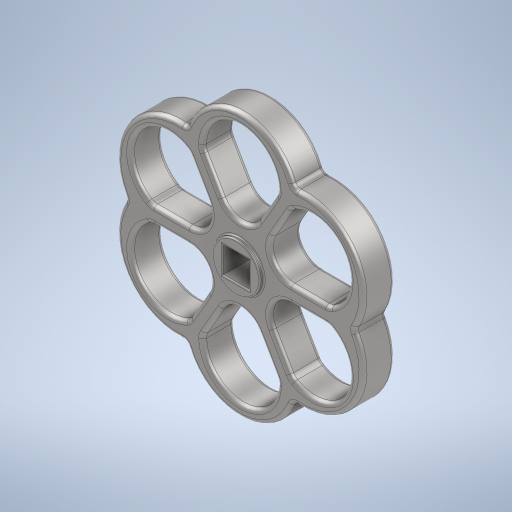
# Autodesk Inventor part: cover 2
Saved by Autodesk Inventor 2024 (Build 280153000, 153)
## iProperties
Created: 2024-04-01
Part Number: cover 2
Material: Generic
Document SubType Name: Modeling
Designer: MSI-C
Density: 1 g/cm^3
Appearance: Stainless - Brushed
Author: MSI-C
Autodesk Inventor part; units mm, degrees
ref_plane "YZ Plane" through (0, 0, 0) normal (1, 0, 0) x (0, 1, 0)
ref_plane "XZ Plane" through (0, 0, 0) normal (0, 1, 0) x (-1, 0, 0)
ref_plane "XY Plane" through (0, 0, 0) normal (0, 0, 1) x (1, 0, 0)
sketch "Sketch1" plane through (0, 0, 0) normal (0, 0, 1) x (1, 0, 0)
  line L0 (-42.5, 0) -> (42.5, 0) construction
  line L1 (0, 0) -> (20, 34.641) construction
  line L2 (0, 0) -> (-20, 34.641) construction
  line L3 (0, 49.3564) -> (0, -48.6436) construction
  arc A0 (19.9086, 34.4827) -> (-20, 34.641) centre (-0.0697, 28.5022) ccw
  line L4 (0, 0) -> (-42.4352, 24.5) construction
  arc A1 (-20, 34.641) -> (-42.5, 0) centre (-23.3657, 12.1995) ccw
  line L5 (0, 0) -> (42.4352, 24.5) construction
  arc A2 (42.5, 0) -> (19.9086, 34.4827) centre (23.5092, 12.1999) ccw
  line L6 (0, 0) -> (20, -34.641) construction
  line L7 (0, 0) -> (-20, -34.641) construction
  line L8 (0, -49.3564) -> (0, 48.6436) construction
  arc A3 (-20, -34.641) -> (19.9086, -34.4827) centre (-0.0697, -28.5022) ccw
  line L9 (0, 0) -> (-42.4352, -24.5) construction
  arc A4 (-42.5, 0) -> (-20, -34.641) centre (-23.3657, -12.1995) ccw
  line L10 (0, 0) -> (42.4352, -24.5) construction
  arc A5 (19.9086, -34.4827) -> (42.5, 0) centre (23.5092, -12.1999) ccw
  dimension "d0" = 85
  dimension "d2" = 60
  dimension "d3" = 60
  dimension "d4" = 98
  dimension "d8" = 30
  dimension "d10" = 30
  dimension "d80" = 22.6925
  dimension "d81" = 22.5719
  dimension "d82" = 20.8543
  dimension "d83" = 22.6925
  dimension "d84" = 20.8543
  dimension "d85" = 22.5719
  dimension "d86" = 34.641
  dimension "d87" = 39.9086
  constraints: 22 end point, 18 point on circle, 10 symmetric about line, 6 centre point, 4 point on line, 2 equal length, 1 horizontal, 1 midpoint, 1 vertical, 3 other
  measures "d0" distance of L0.start L0.end
  measures "d2" angle of L0 L1
  measures "d3" angle of L0 L2
  measures "d4" distance of L3.start L3.end
  measures "d8" angle of L0 L4
  measures "d10" angle of L0 L5
  measures "d80" radius of A1
  measures "d81" radius of A2
  measures "d82" radius of A0
  measures "d83" radius of A4
  measures "d84" radius of A3
  measures "d85" radius of A5
  measures "d86" vertical distance of L0.start L2.end
  measures "d87" horizontal distance of L2.end A0.start
extrude "Extrusion1" add sketch "Sketch1" along normal mid plane 12
sketch "Sketch3" plane through (0, 0, 6) normal (0, 0, 1) x (1, 0, 0)
  line L0 (-64.5205, 0) -> (64.5205, 0) construction
  arc A0 (13.943, 31.2916) -> (-14.0462, 31.5464) centre (-0.0549, 31.0509) ccw
  line L1 (-13.5128, 29.4048) -> (-6.9282, 18)
  line L2 (13.4077, 29.2228) -> (6.9282, 18)
  line L3 (19.9086, 34.4827) -> (0, 0) construction
  line L4 (-20, 34.641) -> (0, 0) construction
  arc A1 (-6.9282, 18) -> (6.9282, 18) centre (0, 22) ccw
  arc A2 (13.4077, 29.2228) -> (13.943, 31.2916) centre (9.9436, 31.2228) ccw
  arc A3 (-14.0462, 31.5464) -> (-13.5128, 29.4048) centre (-10.0487, 31.4048) ccw
  arc A4 (34.0708, 3.5708) -> (20.2969, 27.9375) centre (26.8634, 15.573) ccw
  line L5 (18.7089, 26.4048) -> (12.1244, 15)
  line L6 (32.0115, 3) -> (19.0526, 3)
  line L7 (39.8172, 0) -> (0, 0) construction
  line L8 (20, 34.641) -> (0, 0) construction
  arc A5 (12.1244, 15) -> (19.0526, 3) centre (19.0526, 11) ccw
  arc A6 (32.0115, 3) -> (34.0708, 3.5708) centre (32.0115, 7) ccw
  arc A7 (20.2969, 27.9375) -> (18.7089, 26.4048) centre (22.173, 24.4048) ccw
  arc A8 (20.1278, -27.7208) -> (34.343, -3.6088) centre (26.9183, -15.4779) ccw
  line L9 (32.2217, -3) -> (19.0526, -3)
  line L10 (18.6038, -26.2228) -> (12.1244, -15)
  line L11 (19.9086, -34.4827) -> (0, 0) construction
  line L12 (40, 0) -> (0, 0) construction
  arc A9 (19.0526, -3) -> (12.1244, -15) centre (19.0526, -11) ccw
  arc A10 (18.6038, -26.2228) -> (20.1278, -27.7208) centre (22.0679, -24.2228) ccw
  arc A11 (34.343, -3.6088) -> (32.2217, -3) centre (32.2217, -7) ccw
  arc A12 (-13.943, -31.2916) -> (14.0462, -31.5464) centre (0.0549, -31.0509) ccw
  line L13 (13.5128, -29.4048) -> (6.9282, -18)
  line L14 (-13.4077, -29.2228) -> (-6.9282, -18)
  line L15 (-19.9086, -34.4827) -> (0, 0) construction
  line L16 (20, -34.641) -> (0, 0) construction
  arc A13 (6.9282, -18) -> (-6.9282, -18) centre (0, -22) ccw
  arc A14 (-13.4077, -29.2228) -> (-13.943, -31.2916) centre (-9.9436, -31.2228) ccw
  arc A15 (14.0462, -31.5464) -> (13.5128, -29.4048) centre (10.0487, -31.4048) ccw
  arc A16 (-34.0708, -3.5708) -> (-20.2969, -27.9375) centre (-26.8634, -15.573) ccw
  line L17 (-18.7089, -26.4048) -> (-12.1244, -15)
  line L18 (-32.0115, -3) -> (-19.0526, -3)
  line L19 (-39.8172, 0) -> (0, 0) construction
  line L20 (-20, -34.641) -> (0, 0) construction
  arc A17 (-12.1244, -15) -> (-19.0526, -3) centre (-19.0526, -11) ccw
  arc A18 (-32.0115, -3) -> (-34.0708, -3.5708) centre (-32.0115, -7) ccw
  arc A19 (-20.2969, -27.9375) -> (-18.7089, -26.4048) centre (-22.173, -24.4048) ccw
  arc A20 (-20.1278, 27.7208) -> (-34.343, 3.6088) centre (-26.9183, 15.4779) ccw
  line L21 (-32.2217, 3) -> (-19.0526, 3)
  line L22 (-18.6038, 26.2228) -> (-12.1244, 15)
  line L23 (-19.9086, 34.4827) -> (0, 0) construction
  line L24 (-40, 0) -> (0, 0) construction
  arc A21 (-19.0526, 3) -> (-12.1244, 15) centre (-19.0526, 11) ccw
  arc A22 (-18.6038, 26.2228) -> (-20.1278, 27.7208) centre (-22.0679, 24.2228) ccw
  arc A23 (-34.343, 3.6088) -> (-32.2217, 3) centre (-32.2217, 7) ccw
  point P0 (0, 6)
  point P1 (13.9125, 30.0972)
  point P2 (-14.0353, 30.3099)
  point P3 (33.0212, 3)
  point P4 (19.2315, 27.3099)
  point P5 (5.1962, 3)
  point P6 (19.1087, -27.0972)
  point P7 (33.2668, -3)
  point P8 (5.1962, -3)
  point P9 (-13.9125, -30.0972)
  point P10 (14.0353, -30.3099)
  point P11 (0, -6)
  point P12 (-33.0212, -3)
  point P13 (-19.2315, -27.3099)
  point P14 (-5.1962, -3)
  point P15 (-19.1087, 27.0972)
  point P16 (-33.2668, 3)
  point P17 (-5.1962, 3)
  dimension "d40" = 8
  dimension "d41" = 4
  dimension "d47" = 3
  dimension "d48" = 3
  dimension "d51" = 360
  dimension "d90" = 14
  constraints: 60 point on circle, 48 end point, 24 centre point, 24 point on line, 6 tangent, 2 coincident, 2 parallel, 1 equal radius, 143 other
  measures "d40" radius of A1
  measures "d41" radius of A2
  measures "d47" distance between parallel lines of L2 L3
  measures "d48" distance between parallel lines of L4 L1
  measures "d90" radius of A8
extrude "Extrusion2" cut sketch "Sketch3" against normal through all
sketch "Sketch9" plane through (0, 0, 0) normal (0, 0, 1) x (1, 0, 0)
  circle A0 centre (0, 0) radius 9
  dimension "d30" = 18
  constraints: 1 centre point, 1 coincident
  measures "d30" diameter of A0
extrude "Extrusion5" add sketch "Sketch9" along normal mid plane 15
sketch "Sketch10" plane through (0, 0, 0) normal (0, 0, 1) x (1, 0, 0)
  line L0 (5, -5) -> (-5, -5)
  line L1 (-5, -5) -> (-5, 5)
  line L2 (-5, 5) -> (5, 5)
  line L3 (5, 5) -> (5, -5)
  line L4 (5, -5) -> (-5, 5) construction
  line L5 (-5, -5) -> (5, 5) construction
  point P0 (0, 0)
  dimension "d33" = 10
  dimension "d34" = 10
  constraints: 12 end point, 2 midpoint, 2 parallel, 1 horizontal, 1 perpendicular
  measures "d33" distance of L0.start L0.end
  measures "d34" distance of L2.end L0.start
extrude "Extrusion6" cut sketch "Sketch10" along normal through all both and the other way through all
fillet "Fillet1" radius 2 6 edges at (19.9086, -34.4827, 0) (42.5, 0, 0) (19.9086, 34.4827, 0) (-20, 34.641, 0) (-42.5, 0, 0) (-20, -34.641, 0)
fillet "Fillet2" radius 1.5 96 edges at (20.2177, 34.9724, -6) (42.4986, 24.402, -6) (42.8385, 0, -6) (42.4986, -24.402, -6) (20.2177, -34.9724, -6) (-0.001, -49.3564, -6) (-20.3002, -35.1146, -6) (-42.499, -24.4006, -6) (-42.8341, 0, -6) (-42.499, 24.4006, -6) (-20.3002, 35.1146, -6) (-0.001, 49.3564, -6) (-20.3002, 35.1146, 6) (-42.499, 24.4006, 6) (-42.8341, 0, 6) (-42.499, -24.4006, 6) (-20.3002, -35.1146, 6) (-0.001, -49.3564, 6) (20.2177, -34.9724, 6) (42.4986, -24.402, 6) (42.8385, 0, 6) (42.4986, 24.402, 6) (20.2177, 34.9724, 6) (-0.001, 49.3564, 6) (-13.9301, 30.4381, -6) (-10.2205, 23.7024, -6) (0, 14, -6) (10.1679, 23.6114, -6) (13.816, 30.2208, -6) (0.0725, 45.0503, -6) (19.3951, 27.2828, -6) (15.4166, 20.7024, -6) (12.1244, 7, -6) (25.532, 3, -6) (33.08, 3.1453, -6) (39.051, 22.4624, -6) (12.1244, -7, -6) (15.3641, -20.6114, -6) (19.2639, -27.0754, -6) (38.9785, -22.588, -6) (33.3252, -3.1552, -6) (25.6371, -3, -6) (-13.816, -30.2208, -6) (-0.0725, -45.0503, -6) (13.9301, -30.4381, -6) (10.2205, -23.7024, -6) (0, -14, -6) (-10.1679, -23.6114, -6) (-33.08, -3.1453, -6) (-39.051, -22.4624, -6) (-19.3951, -27.2828, -6) (-15.4166, -20.7024, -6) (-12.1244, -7, -6) (-25.532, -3, -6) (-33.3252, 3.1552, -6) (-25.6371, 3, -6) (-12.1244, 7, -6) (-15.3641, 20.6114, -6) (-19.2639, 27.0754, -6) (-38.9785, 22.588, -6) (-12.1244, 7, 6) (-25.6371, 3, 6) (-33.3252, 3.1552, 6) (-38.9785, 22.588, 6) (-19.2639, 27.0754, 6) (-15.3641, 20.6114, 6) (13.816, 30.2208, 6) (10.1679, 23.6114, 6) (0, 14, 6) (-10.2205, 23.7024, 6) (-13.9301, 30.4381, 6) (0.0725, 45.0503, 6) (33.08, 3.1453, 6) (25.532, 3, 6) (12.1244, 7, 6) (15.4166, 20.7024, 6) (19.3951, 27.2828, 6) (39.051, 22.4624, 6) (19.2639, -27.0754, 6) (15.3641, -20.6114, 6) (12.1244, -7, 6) (25.6371, -3, 6) (33.3252, -3.1552, 6) (38.9785, -22.588, 6) (10.2205, -23.7024, 6) (13.9301, -30.4381, 6) (-0.0725, -45.0503, 6) (-13.816, -30.2208, 6) (-10.1679, -23.6114, 6) (0, -14, 6) (-15.4166, -20.7024, 6) (-19.3951, -27.2828, 6) (-39.051, -22.4624, 6) (-33.08, -3.1453, 6) (-25.532, -3, 6) (-12.1244, -7, 6)
fillet "Fillet3" radius 0.5 12 edges at (-9, 0, -6) (-9, 0, -7.5) (-9, 0, 6) (-9, 0, 7.5) (0, 5, 7.5) (-5, 0, 7.5) (0, -5, 7.5) (5, 0, 7.5) (5, 0, -7.5) (0, -5, -7.5) (-5, 0, -7.5) (0, 5, -7.5)
sketch "Sketch11" plane through (-18.6038, 26.2228, -4.5) normal (-0.866, -0.5, 0) x (0, 0, 1)
  point P0 (4.5, -32.0115)
sketch "Sketch12" plane through (0, 0, -6) normal (0, 0, -1) x (-1, 0, 0)
  point P0 (0, 0)
body "Solid1"
